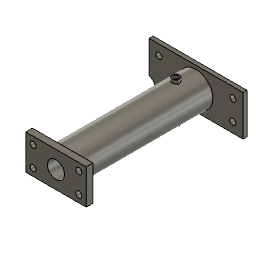
Measurement+Tube+Front+Adapter (Autodesk Fusion 360 design; units mm, degrees)
Autodesk Fusion 360 part; units mm, degrees
note: some values were not read from the file. Set by a fixed rule: which sketch regions a step uses.
sketch "Sketch1" plane through (0, 0, 0) normal (0, 0, 1) x (1, 0, 0)
  circle A0 centre (0, 0) radius 7
  circle A1 centre (0, 0) radius 12.5
  dimension "d1" = 25
  dimension "d2" = 14
  constraint coincident A0.centre A1.centre
  measures "d1" diameter of A1
  measures "d2" diameter of A0
extrude "Extrude1" add sketch "Sketch1" along normal blind 15 contours A0 | A1
sketch "Sketch2" plane through (0, 0, 15) normal (0, 0, 1) x (1, 0, 0)
  circle A0 centre (0, 0) radius 12.5
  circle A1 centre (0, 0) radius 6.375
  dimension "d5" = 12.75
  constraint concentric A0 A1
  measures "d5" diameter of A1
loft "Loft1" cut profiles "Sketch1", "Sketch2" section 1 contours A0 section 2 contours A1
extrude "Extrude2" add 1 faces at (10.4118, -0.621, 15) along direction (0, 0, 1) blind 92
sketch "Sketch17" plane through (0, 0, 107) normal (0, 0, 1) x (1, 0, 0)
  circle A0 centre (-17, -7.5) radius 2.25
  circle A1 centre (17, -7.5) radius 2.25
  circle A2 centre (0, 0) radius 6.375
  circle A3 centre (0, 0) radius 12.5
  line L0 (-22.5, 13) -> (22.5, 13)
  line L1 (22.5, 13) -> (22.5, -13)
  line L2 (22.5, -13) -> (-22.5, -13)
  line L3 (-22.5, -13) -> (-22.5, 13)
  line L4 (0, 0) -> (-22.5, 0) construction
  line L5 (0, 0) -> (22.5, 0) construction
  circle A4 centre (-17, 7.5) radius 2.25
  circle A5 centre (17, 7.5) radius 2.25
  point P0 (-12.5, 0)
  point P1 (12.5, 0)
  dimension "d112" = 4.5
  dimension "d113" = 4.5
  dimension "d147" = 10
  dimension "d148" = 10
  dimension "d149" = 7.5
  dimension "d150" = 13
  dimension "d151" = 17
  dimension "d152" = 17
  dimension "d153" = 7.5
  dimension "d154" = 17
  dimension "d155" = 7.5
  dimension "d156" = 4.5
  dimension "d157" = 4.5
  dimension "d158" = 17
  dimension "d159" = 7.5
  constraint horizontal L0
  constraint vertical L1
  constraint horizontal L2
  constraint vertical L3
  constraint coincident A2.centre A3.centre
  constraint midpoint L3 L4.end
  constraint midpoint L1 L5.end
  constraint horizontal L4
  constraint coincident A3 P0
  constraint coincident L4 P0
  constraint coincident L5 P1
  constraint coincident A3 P1
  measures "d112" diameter of A0
  measures "d113" diameter of A1
  measures "d147" distance of L4.end P0
  measures "d148" distance of L5.end P1
  measures "d149" distance of A0.centre L4
  measures "d150" distance of L2 L4
  measures "d151" horizontal distance of A0.centre A2.centre
  measures "d152" horizontal distance of A1.centre A2.centre
  measures "d153" distance of A1.centre L5
  measures "d154" horizontal distance of A2.centre A4.centre
  measures "d155" distance of L4 A4.centre
  measures "d156" diameter of A4
  measures "d157" diameter of A5
  measures "d158" horizontal distance of A2.centre A5.centre
  measures "d159" distance of L5 A5.centre
extrude "Extrude15" add sketch "Sketch17" against normal blind 5 contours A3 | L0 L1 L2 L3
sketch "Sketch18" plane through (0, 0, 0) normal (0, 0, -1) x (-1, 0, 0)
  circle A0 centre (-17, -7.5) radius 2.25
  circle A1 centre (17, -7.5) radius 2.25
  line L0 (-34.9564, 15) -> (34.9564, 15)
  line L1 (34.9564, 15) -> (34.9564, -15)
  line L2 (34.9564, -15) -> (-34.9564, -15)
  line L3 (-34.9564, -15) -> (-34.9564, 15)
  circle A2 centre (-27.4564, -7.5) radius 2.25
  circle A3 centre (0, 0) radius 7
  circle A4 centre (0, 0) radius 12.5
  line L4 (-22.5, -13) -> (22.5, -13)
  line L5 (22.5, -13) -> (22.5, 13)
  line L6 (22.5, 13) -> (-22.5, 13)
  line L7 (-22.5, 13) -> (-22.5, -13)
  circle A5 centre (0, 0) radius 12.5
  circle A6 centre (-17, 7.5) radius 2.25
  circle A7 centre (17, 7.5) radius 2.25
  circle A8 centre (-27.4564, 7.5) radius 2.25
  circle A9 centre (27.4564, 7.5) radius 2.25
  point P0 (0, -15)
  dimension "d122" = 4.5
  dimension "d124" = 7.5
  dimension "d125" = 7.5
  dimension "d160" = 34.9564
  dimension "d161" = 15
  dimension "d162" = 34.9564
  dimension "d163" = 15
  dimension "d164" = 7.5
  dimension "d165" = 7.5
  dimension "d166" = 4.5
  dimension "d167" = 7.5
  dimension "d168" = 7.5
  dimension "d169" = 4.5
  constraint horizontal L0
  constraint vertical L1
  constraint horizontal L2
  constraint vertical L3
  constraint midpoint L2 P0
  measures "d122" diameter of A2
  measures "d124" distance of L2 A2.centre
  measures "d125" distance of L3 A2.centre
  measures "d160" distance of A3.centre L3
  measures "d161" distance of A3.centre L2
  measures "d162" distance of L1.end P0
  measures "d163" distance of A3.centre L0
  measures "d164" distance of L0 A8.centre
  measures "d165" distance of L3 A8.centre
  measures "d166" diameter of A8
  measures "d167" distance of L1 A9.centre
  measures "d168" distance of L0 A9.centre
  measures "d169" diameter of A9
extrude "Extrude16" add sketch "Sketch18" against normal blind 3 contours A0 | A1 | L0 L1 L2 L3 | L4 L5 L6 L7 | A6 | A7
ref_plane "WorkPlane5" through (0, -7, 0) normal (0, 1, 0) x (0, 0, 1)
sketch "Sketch19" plane through (0, -7, 0) normal (0, 1, 0) x (1, 0, 0)
  line L0 (6.375, -15) -> (-6.375, -15)
  line L1 (0, -15) -> (0, -107) construction
  circle A0 centre (0, -18) radius 1.7
  circle A1 centre (0, -18) radius 2.7
  line L2 (6.375, -107) -> (-6.375, -107)
  dimension "d131" = 3.4
  dimension "d132" = 5.4
  dimension "d139" = 3
  constraint midpoint L0 L1.start
  constraint concentric A0 A1
  constraint coincident L1 A0.centre
  constraint midpoint L1.end L2
  measures "d131" diameter of A0
  measures "d132" diameter of A1
  measures "d139" distance of L0 A0.centre
extrude "Extrude17" add sketch "Sketch19" against normal blind 8
extrude "Extrude18" cut sketch "Sketch19" along normal blind 2 and the other way blind 8 contours A0
ref_plane "WorkPlane7" through (0, 7, 0) normal (0, 1, 0) x (0, 0, 1)
sketch "Sketch22" plane through (0, 7, 0) normal (0, 1, 0) x (1, 0, 0)
  circle A0 centre (0, -18) radius 1.7
  circle A1 centre (0, -18) radius 2.7
  point P0 (0, -18)
  dimension "d171" = 3.4
  dimension "d172" = 5.4
  constraint coincident P0 A0.centre
  measures "d171" diameter of A0
  measures "d172" diameter of A1
extrude "Extrude21" add sketch "Sketch22" along normal blind 8
extrude "Extrude22" cut sketch "Sketch22" along normal blind 8 and the other way blind 2 contours A0
sketch "Sketch23" plane through (0, 0, 0) normal (0, 0, -1) x (-1, 0, 0)
  line L0 (-34.9564, -15) -> (34.9564, -15)
  line L1 (34.9564, -15) -> (34.9564, 15)
  line L2 (34.9564, 15) -> (-34.9564, 15)
  line L3 (-34.9564, 15) -> (-34.9564, -15)
  circle A0 centre (-27.4564, 7.5) radius 2.25
  circle A1 centre (-27.4564, -7.5) radius 2.25
  circle A2 centre (27.4564, 7.5) radius 2.25
  circle A3 centre (0, 0) radius 7
  line L4 (34.9564, -15) -> (30.1724, -15)
  line L5 (34.9564, -9.125) -> (34.9564, -15)
  arc A4 (34.9564, -9.125) -> (30.1724, -15) centre (36.8966, -15.5902) ccw
  dimension "d181" = 4.784
  dimension "d182" = 5.875
  dimension "d183" = 6.75
  constraint horizontal L4
  constraint vertical L5
  constraint coincident L0.end L1.start
  measures "d181" distance of L0.end L4.end
  measures "d182" distance of L0.end L5.start
  measures "d183" radius of A4
extrude "Extrude23" cut sketch "Sketch23" against normal up to surface (3 mm away) contours L0 L1 L4 L5 A4
equation "d110 = 15 mm"
equation "d113 = d112"
equation "d116 = d110 / 2"
equation "d125 = d124"
equation "d130 = -d2 / 2"
equation "d132 = d131 + 2 mm"
equation "d148 = d147"
equation "d152 = d151"
equation "d153 = d149"
equation "d154 = d151"
equation "d155 = d149"
equation "d156 = d112"
equation "d157 = d112"
equation "d158 = d151"
equation "d159 = d149"
equation "d162 = d160"
equation "d163 = d161"
equation "d164 = d124"
equation "d165 = d124"
equation "d166 = d122"
equation "d167 = d124"
equation "d168 = d124"
equation "d169 = d122"
equation "d170 = ( d2 / 2 mm ) * 1 mm"
equation "d172 = d171 + 2 mm"
equation "d64 = d67"
equation "d67 = 40.00 mm"
equation "d70 = d67"
equation "d82 = -d67"
equation "d96 = d26 / 2"
equation "d97 = d16 / 2"
equation "d101 = -d29"
equation "d105 = -d29"
equation "d114 = 17 mm"
equation "d115 = d114"
equation "d117 = d116"
equation "d126 = d124"
equation "d127 = d124"
